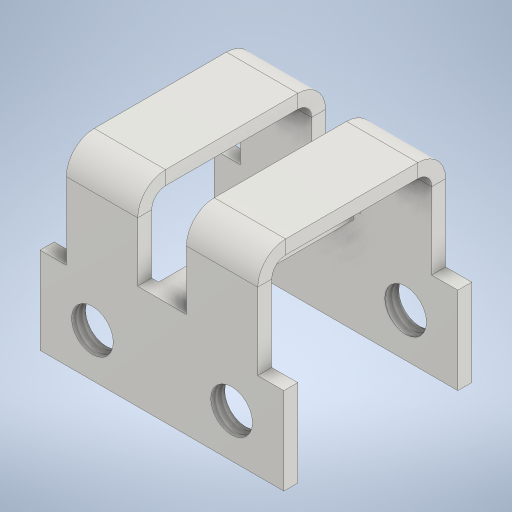
# Autodesk Inventor part: Encaixe Macaco
Saved by Autodesk Inventor 2024 (Build 280153000, 153)
## iProperties
Created: 2024-06-03
Part Number: Encaixe Macaco
Material: Steel AISI 1050
Document SubType Name: Sheet Metal
Designer: Pedro
Density: 7.85 g/cm^3
Sheet Metal Rule: Default_mm
Appearance: Steel
Mass: 268.625 g
Surface Area: 215.337 cm^2
Volume: 34.2198 cm^3
Author: Pedro
Autodesk Inventor part; units mm, degrees
ref_plane "YZ Plane" through (0, 0, 0) normal (1, 0, 0) x (0, 1, 0)
ref_plane "XZ Plane" through (0, 0, 0) normal (0, 1, 0) x (-1, 0, 0)
ref_plane "XY Plane" through (0, 0, 0) normal (0, 0, 1) x (1, 0, 0)
sketch "Sketch1" plane through (0, 0, 0) normal (0, 0, 1) x (1, 0, 0)
  line L0 (51.3286, 13.0104) -> (51.3286, -6.9896)
  line L1 (51.3286, -6.9896) -> (51.3286, -16.9896)
  line L2 (51.3286, -16.9896) -> (58.8286, -16.9896)
  line L3 (58.8286, -16.9896) -> (58.8286, -41.9896)
  line L4 (58.8286, -41.9896) -> (-11.1714, -41.9896)
  line L5 (-11.1714, -41.9896) -> (-11.1714, -16.9896)
  line L6 (-11.1714, -16.9896) -> (-3.6714, -16.9896)
  line L7 (-3.6714, -16.9896) -> (-3.6714, -6.9896)
  line L8 (-3.6714, -6.9896) -> (-3.6714, 13.0104)
  line L9 (16.8286, 8.0104) -> (16.8286, -11.9896)
  line L10 (16.8286, -11.9896) -> (30.8286, -11.9896)
  line L11 (30.8286, -11.9896) -> (30.8286, 8.0104)
  line L12 (-3.6714, 13.0104) -> (51.3286, 13.0104)
  line L13 (16.8286, 8.0104) -> (16.8286, 13.0104)
  line L14 (30.8286, 8.0104) -> (30.8286, 13.0104)
  point P0 (0, 0)
  dimension "d1" = 20
  dimension "d2" = 10
  dimension "d3" = 7.5
  dimension "d4" = 25
  dimension "d5" = 70
  dimension "d7" = 20
  dimension "d8" = 14
  dimension "d93" = 25
  measures "d1" distance of L0.start L0.end
  measures "d2" distance of L0.end L1.end
  measures "d3" distance of L1.end L2.end
  measures "d4" distance of L2.end L3.end
  measures "d5" distance of L3.end L4.end
  measures "d7" distance of L9.start L9.end
  measures "d8" distance of L9.end L10.end
  measures "d93" distance from line of L10 L13.end
extrude "Plate1" add sketch "Sketch1" along normal blind 4 contours L0 L1 L2 L3 L4 L5 L6 L7 L8 L12 L13 L9 L10 L11 L14
sketch "Sketch2" plane through (16.8286, 9.0104, 4) normal (0, 1, 0) x (-1, 0, 0)
  line L0 (20.5, 0) -> (0, 0)
  line L1 (0, 0) -> (0, -27)
  line L2 (0, -27) -> (20.5, -27)
  line L3 (20.5, -27) -> (20.5, 0)
  constraints: 6 end point, 1 horizontal, 1 perpendicular, 1 vertical
edge flange "Flange1" height 27 angle 90 thickness 4 bend radius 4 thickness toward (0, 1, 0) relief straight relief width 4 relief depth 2 corner gap 4 corner form 0 edges at (6.5786, 13.0104, 0) (41.0786, 13.0104, 0) wall of the first edge with corners at (-3.6714, 9.0104, 4) (16.8286, 9.0104, 4) (16.8286, 9.0104, -23) (-3.6714, 9.0104, -23)
bend "Bend1"
corner "Corner1"
ref_plane "Work Plane2" through (0, 0, -23) normal (0, 0, 1) x (1, 0, 0)
mirror "Mirror1" about plane through (0, 0, -23) normal (0, 0, 1) of "Plate1"
sketch "Sketch6" plane through (-3.6714, 9.0104, -50) normal (0, 1, 0) x (-1, 0, 0)
  line L0 (-20.5, 0) -> (0, 0)
  line L1 (0, 0) -> (0, 27)
  line L2 (0, 27) -> (-20.5, 27)
  line L3 (-20.5, 27) -> (-20.5, 0)
  constraints: 6 end point, 1 horizontal, 1 perpendicular, 1 vertical
edge flange "Flange4" height 27 angle 90 thickness 4 bend radius 4 thickness toward (0, 1, 0) relief straight relief width 4 relief depth 2 corner gap 4 corner form 0 edges at (6.5786, 13.0104, -46) (41.0786, 13.0104, -46) wall of the first edge with corners at (16.8286, 9.0104, -50) (-3.6714, 9.0104, -50) (-3.6714, 9.0104, -23) (16.8286, 9.0104, -23)
bend "Bend4"
corner "Corner4"
sketch "Sketch7" plane through (0, 0, 4) normal (0, 0, 1) x (1, 0, 0)
  circle A0 centre (3.8286, -29.4896) radius 6
  circle A1 centre (43.8286, -29.4896) radius 6
  line L0 (16.8286, -11.9896) -> (30.8286, -11.9896) projected
  line L1 (58.8286, -41.9896) -> (-11.1714, -41.9896) projected
  line L2 (51.3286, -16.9896) -> (58.8286, -16.9896) projected
  point P0 (0, 0)
  point P1 (23.8286, -11.9896)
  dimension "d55" = 12
  dimension "d56" = 12
  dimension "d57" = 40
  dimension "d58" = 20
  dimension "d59" = 12.5
  dimension "d60" = 12.5
  constraints: 2 centre point, 1 midpoint
  measures "d55" diameter of A0
  measures "d56" diameter of A1
  measures "d57" distance of A1.centre A0.centre
  measures "d58" horizontal distance of A0.centre point (23.829, -11.99)
  measures "d59" distance from line of L1 A0.centre
  measures "d60" distance from line of L2 A1.centre
extrude "Extrusion1" cut sketch "Sketch7" against normal blind 80
thread "Thread1" size "M12x1.75" class "6H" standard "ANSI Metric M Profile" full length
thread "Thread2" size "M12x1.75" class "6H" standard "ANSI Metric M Profile" full length
thread "Thread3" size "M12x1.75" class "6H" standard "ANSI Metric M Profile" full length
thread "Thread4" size "M12x1.75" class "6H" standard "ANSI Metric M Profile" full length
sketch "Sketch10" plane through (-11.1714, -41.9896, -46) normal (0, 0, 1) x (1, 0, 0)
  line L0 (42, 30) -> (28, 30) projected
  line L1 (30, 30) -> (40, 30)
  line L2 (40, 30) -> (40, 27.5)
  line L3 (40, 27.5) -> (30, 27.5)
  line L4 (30, 27.5) -> (30, 30)
  point P0 (11.1714, 41.9896)
  point P1 (35, 30)
  dimension "d94" = 10
  dimension "d95" = 2.5
  dimension "d96" = 7
  constraints: 8 end point, 2 parallel, 2 point on line, 1 midpoint, 1 perpendicular
  measures "d94" distance of L1.start L1.end
  measures "d95" distance of L3.end L1.start
  measures "d96" distance of L0.end point (35, 30)
extrude "Extrusion2" add sketch "Sketch10" along normal up to surface (46 mm away)
equation "\"d12\" = Thickness"
equation "\"d13\" = BendReliefWidth"
equation "\"d14\" = BendReliefDepth"
equation "\"d15\" = MinimumRemnant"
equation "\"d16\" = TransitionRadius"
equation "\"d19\" = BendRadius"
equation "\"d20\" = CornerReliefSize"
equation "\"d21\" = GapSize"
equation "\"d22\" = JacobiRadiusSize"
equation "\"d45\" = BendReliefWidth"
equation "\"d46\" = BendReliefDepth"
equation "\"d47\" = MinimumRemnant"
equation "\"d48\" = TransitionRadius"
equation "\"d51\" = BendRadius"
equation "\"d52\" = CornerReliefSize"
equation "\"d53\" = GapSize"
equation "\"d54\" = JacobiRadiusSize"
equation "\"BendRadius\" = Thickness"
equation "\"BendReliefWidth\" = Thickness"
equation "\"BendReliefDepth\" = 0.5 * Thickness"
equation "\"CornerReliefSize\" = 4 * Thickness"
equation "\"MinimumRemnant\" = 2 * Thickness"
equation "\"TransitionRadius\" = BendRadius"
equation "\"JacobiRadiusSize\" = BendRadius"
equation "\"GapSize\" = Thickness"
equation "\"Thickness\" = 4"
body "Solid1"
